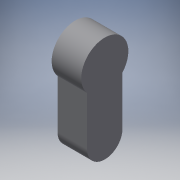
# Autodesk Inventor part: OtherCamera
Saved by Autodesk Inventor 2017 (Build 210142000, 142)
## iProperties
Created: 2017-02-18
Part Number: OtherCamera
Material: Generic
Document SubType Name: Modeling
Designer: Roksbot
Density: 1 g/cm^3
Appearance: Default
Author: Roksbot
Autodesk Inventor part; units mm, degrees
ref_plane "YZ Plane" through (0, 0, 0) normal (1, 0, 0) x (0, 1, 0)
ref_plane "XZ Plane" through (0, 0, 0) normal (0, 1, 0) x (-1, 0, 0)
ref_plane "XY Plane" through (0, 0, 0) normal (0, 0, 1) x (1, 0, 0)
sketch "Sketch1" plane through (0, 0, 0) normal (1, 0, 0) x (0, 1, 0)
  circle A0 centre (-127.5274, 0) radius 19.939
  line L0 (-73.0444, 0) -> (-182.0104, 0) construction
  line L1 (-140.6798, 14.986) -> (-182.0104, 14.986)
  line L2 (-182.0104, -14.986) -> (-140.6798, -14.986)
  arc A1 (-182.0104, 14.986) -> (-182.0104, -14.986) centre (-182.0104, 0) ccw
  point P0 (0, 0)
  dimension "d0" = 39.878
  dimension "d1" = 29.972
  dimension "d2" = 89.408
  constraints: 8 end point, 4 point on circle, 2 centre point, 2 horizontal, 2 tangent, 1 horizontal alignment, 1 midpoint, 1 parallel, 1 other
  measures "d0" diameter of A0
  measures "d1" distance between parallel lines of L1 L2
extrude "Extrusion1" add sketch "Sketch1" along normal blind 25.019
body "Solid1"
